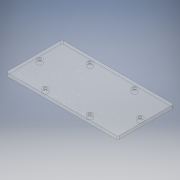
# Autodesk Inventor part: BT004_trajan20_21
Saved by Autodesk Inventor 2022.2 (Build 262287000, 287)
## iProperties
Company: HTBLA Kaindorf
RuleStatus: InUse
Created: 2022-08-07
Part Number: BT004_trajan20_21
Project: Zeichenmaschine_v2
Material: Acryl
Description: Hauptplatte unten
Document SubType Name: Modeling
Designer: trajan20
Density: 1.188 g/cm^3
Appearance: Transparent - farblos
Mass: 139.411 g
Surface Area: 443.675 cm^2
Volume: 117.349 cm^3
AfterDocNew0: iProperties-Editor_aufrufen
Author: jan
Keywords: 2021
Autodesk Inventor part; units mm, degrees
ref_plane "YZ Plane" through (0, 0, 0) normal (1, 0, 0) x (0, 1, 0)
ref_plane "XZ Plane" through (0, 0, 0) normal (0, 1, 0) x (-1, 0, 0)
ref_plane "XY Plane" through (0, 0, 0) normal (0, 0, 1) x (1, 0, 0)
sketch "Skizze4" plane through (0, 0, 0) normal (0, 0, 1) x (1, 0, 0)
  line L0 (0, 0) -> (-100, 0)
  line L1 (-100, 0) -> (-100, 200)
  line L2 (-100, 200) -> (0, 200)
  line L3 (0, 200) -> (0, 0)
  line L4 (-50, 22.6255) -> (-50, -31.1035) construction
  line L5 (-111.0989, 60) -> (-81.531, 60) construction
  point P0 (-50, 10)
  point P1 (-90, 60)
  point P2 (-50, 0)
  dimension "d6" = 100
  dimension "d7" = 200
  dimension "d20" = 10
  dimension "d21" = 10
  dimension "d31" = 60
  constraints: 12 end point, 3 perpendicular, 3 point on line, 2 horizontal, 2 parallel, 1 midpoint, 1 vertical
  measures "d6" distance between parallel lines of L1 L3
  measures "d7" distance between parallel lines of L2 L0
  measures "d20" distance from line of point (-90, 60) L1
  measures "d21" distance from line of L0 point (-50, 10)
  measures "d31" distance between parallel lines of L0 L5
extrude "Extrusion3" add sketch "Skizze4" along normal blind 6
hole "Bohrung1" at (-50, 10, 0) at (-90, 60, 0) direction (0, 0, 1) diameter 5.5 end through all counterbore diameter 10 counterbore depth 5.4
ref_plane "Arbeitsebene1" through (0, 100, 0) normal (0, -1, 0) x (1, 0, 0)
ref_plane "Arbeitsebene2" through (-50, 200, 0) normal (-1, 0, 0) x (0, -1, 0)
mirror "Spiegeln1" about plane through (0, 100, 0) normal (0, -1, 0) of "Bohrung1"
mirror "Spiegeln2" about plane through (-50, 200, 0) normal (-1, 0, 0) of "Spiegeln1", "Bohrung1"
fillet "Rundung2" radius 2 4 edges at (0, 0, 3) (-100, 0, 3) (-100, 200, 3) (0, 200, 3)
